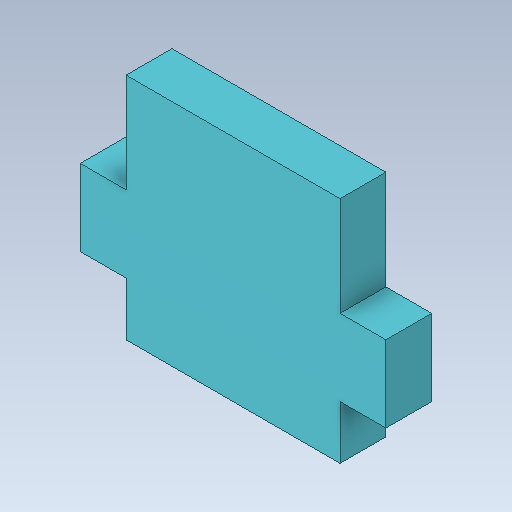
# Autodesk Inventor part: abajo
Saved by Autodesk Inventor 2020 (Build 240168000, 168)
## iProperties
Created: 2020-03-13
Part Number: abajo
Material: Genérico
Document SubType Name: Modeling
Designer: joser
Density: 1 g/cm^3
Appearance: Azul cadete
Author: joser
Autodesk Inventor part; units mm, degrees
ref_plane "YZ Plane" through (0, 0, 0) normal (1, 0, 0) x (0, 1, 0)
ref_plane "XZ Plane" through (0, 0, 0) normal (0, 1, 0) x (-1, 0, 0)
ref_plane "XY Plane" through (0, 0, 0) normal (0, 0, 1) x (1, 0, 0)
sketch "Boceto2" plane through (0, 0, 0) normal (0, 0, 1) x (1, 0, 0)
  line L0 (-14, 15) -> (0, 15)
  line L1 (3, 8.5) -> (3, 3.5)
  line L2 (0, 0) -> (-14, 0)
  line L3 (-17, 3.5) -> (-17, 8.5)
  line L4 (-14, 8.5) -> (-17, 8.5)
  line L5 (-17, 3.5) -> (-14, 3.5)
  line L6 (0, 8.5) -> (3, 8.5)
  line L7 (0, 3.5) -> (3, 3.5)
  line L8 (-14, 15) -> (-14, 8.5)
  line L9 (-14, 3.5) -> (-14, 0)
  line L10 (0, 15) -> (0, 8.5)
  line L11 (0, 3.5) -> (0, 0)
  point P0 (1.5, 3.5)
  dimension "d4" = 20
  dimension "d5" = 15
  dimension "d9" = 5
  dimension "d10" = 3
  dimension "d11" = 3
  dimension "d12" = 5
  dimension "d15" = 3.5
  constraints: 24 end point, 5 parallel, 5 perpendicular, 3 horizontal, 1 coincident, 1 midpoint, 1 point on line, 1 vertical
  measures "d4" distance between parallel lines of L1 L3
  measures "d5" distance between parallel lines of L2 L0
  measures "d9" distance of L3.start L3.end
  measures "d10" distance between parallel lines of L9 L3
  measures "d11" distance from line of L1.end L11
  measures "d12" distance of L1.start L1.end
  measures "d15" distance between parallel lines of L2 L5
extrude "Extrusión1" add sketch "Boceto2" along normal blind 3
